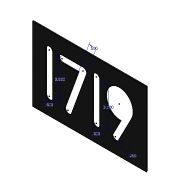
# Autodesk Inventor part: Number Plate
Saved by Autodesk Inventor 2015 (Build 190159000, 159)
## iProperties
Created: 2015-01-25
Part Number: Number Plate
Material: Generic
Document SubType Name: Sheet Metal
Designer: Peter
Density: 1 g/cm^3
Sheet Metal Rule: Default
Appearance: Black Cast
Author: Peter
Autodesk Inventor part; units mm, degrees
ref_plane "YZ Plane" through (0, 0, 0) normal (1, 0, 0) x (0, 1, 0)
ref_plane "XZ Plane" through (0, 0, 0) normal (0, 1, 0) x (-1, 0, 0)
ref_plane "XY Plane" through (0, 0, 0) normal (0, 0, 1) x (1, 0, 0)
sketch "Sketch1" plane through (0, 0, 0) normal (0, 0, 1) x (1, 0, 0)
  line L0 (0, 0) -> (215.9, 0)
  line L1 (215.9, 0) -> (215.9, 139.7)
  line L2 (215.9, 139.7) -> (0, 139.7)
  line L3 (0, 139.7) -> (0, 0)
  dimension "d0" = 215.9
  dimension "d1" = 139.7
  measures "d0" distance of L2.end L1.end
  measures "d1" distance of L1.end L0.end
extrude "Plate1" add sketch "Sketch1" along normal blind 2.286
sketch "Sketch2" plane through (0, 0, 2.286) normal (0, 0, 1) x (1, 0, 0)
  line L0 (0, 0) -> (0, 139.7) projected
  line L1 (215.9, 0) -> (0, 0) projected
  line L2 (215.9, 139.7) -> (215.9, 0) projected
  line L3 (0, 139.7) -> (215.9, 139.7) projected
sketch "Sketch3" plane through (0, 0, 2.286) normal (0, 0, 1) x (1, 0, 0)
  line L0 (0, 0) -> (0, 139.7)
  line L1 (215.9, 0) -> (0, 0)
  line L2 (215.9, 139.7) -> (215.9, 0)
  line L3 (0, 139.7) -> (215.9, 139.7)
  line L4 (38.1, 108.0084) -> (38.1, 31.8084)
  line L5 (25.4, 31.8084) -> (25.4, 108.0084)
  arc A0 (38.1, 108.0084) -> (25.4, 108.0084) centre (31.75, 108.0084) ccw
  arc A1 (25.4, 31.8084) -> (38.1, 31.8084) centre (31.75, 31.8084) ccw
  line L6 (127.1585, 108.0084) -> (127.1585, 31.8084)
  line L7 (114.4585, 31.8084) -> (114.4585, 108.0084)
  arc A2 (127.1585, 108.0084) -> (114.4585, 108.0084) centre (120.8085, 108.0084) ccw
  arc A3 (114.4585, 31.8084) -> (127.1585, 31.8084) centre (120.8085, 31.8084) ccw
  line L8 (55.9503, 111.8766) -> (95.9974, 111.8766)
  line L9 (102.0898, 103.1902) -> (73.5837, 24.4878)
  line L10 (55.9503, 99.1766) -> (87.1287, 99.1766)
  line L11 (87.1287, 99.1766) -> (61.6428, 28.8128)
  line L12 (73.5837, 24.4878) -> (73.5837, 24.4878)
  arc A4 (55.9503, 111.8766) -> (55.9503, 99.1766) centre (55.9503, 105.5266) ccw
  arc A5 (61.6428, 28.8128) -> (73.5837, 24.4878) centre (67.6132, 26.6503) ccw
  arc A6 (102.0898, 103.1902) -> (95.9974, 111.8766) centre (95.9974, 105.3969) ccw
  ellipse E0 centre (164.6613, 85.8797) end of major axis (164.6613, 113.2513) minor radius 25.8041 (187.1505, 72.4584) -> (166.8072, 58.6028) ccw
  line L13 (187.1505, 72.4584) -> (162.6138, 25.1653)
  arc A7 (150.6572, 27.4744) -> (162.6138, 25.1653) centre (156.9773, 28.0896) ccw
  line L14 (150.6572, 27.4744) -> (166.8072, 58.6028)
  dimension "d15" = 12.7
  dimension "d16" = 76.2
  dimension "d17" = 12.7
  dimension "d18" = 76.2
  dimension "d19" = 12.7
  dimension "d33" = 6.35
  constraints: 30 end point, 16 point on circle, 8 centre point, 1 point on line, 5 other
  measures "d15" distance of L4.end L5.start
  measures "d16" distance of L4.start L4.end
  measures "d17" distance of L6.end L7.start
  measures "d18" distance of L6.start L6.end
  measures "d19" distance between parallel lines of L9 L11
  measures "d33" radius of A7
extrude "Cut2" cut sketch "Sketch3" against normal blind 2.286 contours L4 A1 L5 A0 | L6 A3 L7 A2 | L8 A6 L9 A5 L11 L10 A4 | L13 A7 L14 E0
sketch "Sketch4" plane through (0, 0, 2.286) normal (0, 0, 1) x (1, 0, 0)
  line L0 (87.1287, 99.1766) -> (55.9503, 99.1766) projected
  arc A0 (55.9503, 111.8766) -> (55.9503, 99.1766) centre (55.9503, 105.5266) ccw projected
  line L1 (55.9503, 111.8766) -> (95.9974, 111.8766) projected
  arc A1 (102.0898, 103.1902) -> (95.9974, 111.8766) centre (95.9974, 105.3969) ccw projected
  line L2 (102.0898, 103.1902) -> (73.5837, 24.4878) projected
  arc A2 (61.6428, 28.8128) -> (73.5837, 24.4878) centre (67.6132, 26.6503) ccw projected
  line L3 (61.6428, 28.8128) -> (87.1287, 99.1766) projected
  arc A3 (25.4, 31.8084) -> (38.1, 31.8084) centre (31.75, 31.8084) ccw projected
  line L4 (25.4, 31.8084) -> (25.4, 108.0084) projected
  arc A4 (38.1, 108.0084) -> (25.4, 108.0084) centre (31.75, 108.0084) ccw projected
  line L5 (38.1, 108.0084) -> (38.1, 31.8084) projected
  arc A5 (114.4585, 31.8084) -> (127.1585, 31.8084) centre (120.8085, 31.8084) ccw projected
  line L6 (114.4585, 31.8084) -> (114.4585, 108.0084) projected
  arc A6 (127.1585, 108.0084) -> (114.4585, 108.0084) centre (120.8085, 108.0084) ccw projected
  line L7 (127.1585, 108.0084) -> (127.1585, 31.8084) projected
  line L8 (150.6572, 27.4744) -> (166.8072, 58.6028) projected
  ellipse E0 centre (164.6613, 85.8797) end of major axis (164.6613, 113.2513) minor radius 25.8041 (187.1505, 72.4584) -> (166.8072, 58.6028) ccw projected
  line L9 (187.1505, 72.4584) -> (162.6138, 25.1653) projected
  arc A7 (150.6572, 27.4744) -> (162.6138, 25.1653) centre (156.9773, 28.0896) ccw projected
  line L10 (0, 0) -> (0, 139.7) projected
  line L11 (215.9, 0) -> (0, 0) projected
  line L12 (215.9, 139.7) -> (215.9, 0) projected
  line L13 (0, 139.7) -> (215.9, 139.7) projected
  constraints: 1 other
equation "\"d36\" = Thickness"
equation "\"BendRadius\" = Thickness"
equation "\"BendReliefWidth\" = Thickness"
equation "\"BendReliefDepth\" = 0.5 * Thickness"
equation "\"CornerReliefSize\" = 4 * Thickness"
equation "\"MinimumRemnant\" = 2 * Thickness"
equation "\"TransitionRadius\" = BendRadius"
equation "\"JacobiRadiusSize\" = BendRadius"
equation "\"GapSize\" = Thickness"
equation "\"d2\" = BendRadius"
equation "\"Thickness\" = 2.286"
body "Solid1"
